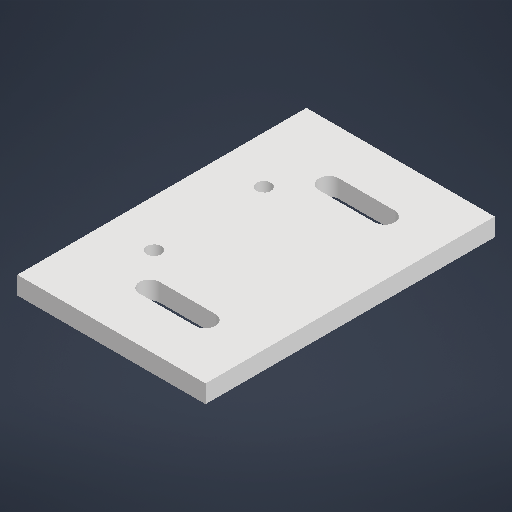
# Autodesk Inventor part: Halterung_Führungsschiene_Version2
Saved by Autodesk Inventor 2027 (Build 310192060, 192F)
## iProperties
Created: 2026-06-12
Part Number: Halterung_Führungsschiene_Version2
Material: Generic
Document SubType Name: Modeling
Designer: kw
Density: 1 g/cm^3
Appearance: Default
Author: kw
Autodesk Inventor part; units mm, degrees
ref_plane "YZ Plane" through (0, 0, 0) normal (1, 0, 0) x (0, 1, 0)
ref_plane "XZ Plane" through (0, 0, 0) normal (0, 1, 0) x (-1, 0, 0)
ref_plane "XY Plane" through (0, 0, 0) normal (0, 0, 1) x (1, 0, 0)
sketch "Sketch1" plane through (0, 0, 0) normal (0, 1, 0) x (-1, 0, 0)
  arc A0 (23.5, 20) -> (23.5, 29) centre (23.5, 24.5) ccw
  line L0 (23.5, 20) -> (-1.5, 20)
  line L1 (23.5, 29) -> (-1.5, 29)
  arc A1 (-1.5, 29) -> (-1.5, 20) centre (-1.5, 24.5) ccw
  arc A2 (23.5, 100) -> (23.5, 109) centre (23.5, 104.5) ccw
  line L2 (23.5, 100) -> (-1.5, 100)
  line L3 (23.5, 109) -> (-1.5, 109)
  arc A3 (-1.5, 109) -> (-1.5, 100) centre (-1.5, 104.5) ccw
  line L4 (74, 129) -> (0, 129)
  line L5 (0, 129) -> (74, 129)
  line L6 (74, 129) -> (74, 0)
  line L7 (74, 0) -> (0, 0)
  line L8 (0, 0) -> (0, 129)
  line L9 (0, 129) -> (-26, 129)
  line L10 (-26, 129) -> (-26, 0)
  line L11 (-26, 0) -> (0, 0)
  line L12 (0, 0) -> (0, 129)
  line L13 (74, 0) -> (58, 0)
  line L14 (58, 0) -> (58, 129)
  line L15 (58, 129) -> (74, 129)
  line L16 (74, 129) -> (74, 0)
  point P0 (0, 0)
  point P1 (23.5, 104.5)
  point P2 (0, 109)
  point P3 (0, 20)
  point P4 (0, 29)
  point P5 (0, 100)
  dimension "d98" = 74
  dimension "d106" = 26
  dimension "d118" = 16
  constraints: 34 end point, 8 point on circle, 6 parallel, 4 centre point, 3 horizontal, 3 perpendicular, 2 point on line
  measures "d98" distance of L4.start L4.end
  measures "d106" distance of L11.end L10.end
  measures "d118" distance of L14.end L15.end
extrude "Extrusion1" add sketch "Sketch1" along normal blind 8 contours A0 L1 L8 L2 A2 L3 L4 L14 L7 L0 | L8 L11 L10 L9 L3 A3 L2 L1 A1 L0
sketch "Sketch4" plane through (0, 0, 0) normal (0, -1, 0) x (1, 0, 0)
  line L0 (-74, 0) -> (-74, 129) projected
  line L1 (-74, 129) -> (0, 0)
  line L2 (0, 100) -> (0, 0) projected
  line L3 (0, 129) -> (-74, 0)
  line L4 (-37, 0) -> (-37, 129)
  line L5 (-58, 129) -> (26, 129) projected
  line L6 (-37, 129) -> (-37, 89)
  line L7 (-37, 129) -> (3, 129) construction
  line L8 (-37, 89) -> (-37, 40)
  line L9 (-37, 40) -> (-37, 0)
  point P0 (-37, 64.5)
  dimension "d119" = 40
  dimension "d120" = 90
  dimension "d121" = 49
  dimension "d122" = 40
  constraints: 14 end point, 2 coincident, 2 collinear, 2 point on line, 1 horizontal, 1 midpoint, 1 perpendicular, 1 vertical
  measures "d119" distance of L4.end L6.end
  measures "d120" angle of L6 L7
  measures "d121" distance of L6.end L8.end
  measures "d122" distance of L8.end L4.start
hole "Hole1" at (-37, 0, 89) at (-37, 0, 40) direction (0, 1, 0) diameter 6.4 depth 20 countersink diameter 12.6 countersink angle 90 clearance for "Countersunk Flat Head Screw ISO 2009/7046" size "M6" standard "ISO"
body "Solid1"
